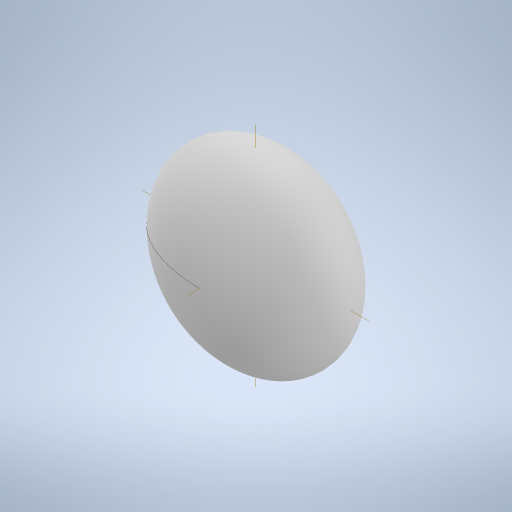
# Autodesk Inventor part: Ellipsoid
Saved by Autodesk Inventor 2023.1 (Build 271208000, 208)
## iProperties
Created: 2023-01-19
Part Number: Ellipsoid
Material: Generisch
Document SubType Name: Modeling
Designer: mehan
Density: 1 g/cm^3
Appearance: Vorgabe
Author: mehan
Autodesk Inventor part; units mm, degrees
ref_plane "YZ Plane" through (0, 0, 0) normal (1, 0, 0) x (0, 1, 0)
ref_plane "XZ Plane" through (0, 0, 0) normal (0, 1, 0) x (-1, 0, 0)
ref_plane "XY Plane" through (0, 0, 0) normal (0, 0, 1) x (1, 0, 0)
sketch "Skizze1" plane through (0, 0, 0) normal (0, 1, 0) x (-1, 0, 0)
  ellipse E0 centre (0, 0) end of major axis (75, 0) minor radius 45 (0, -45) -> (0, 45) ccw
  line L0 (0, 45) -> (0, -45)
  line L1 (0, 0) -> (75, 0) construction
  dimension "d4" = 90
  dimension "d5" = 75
  constraints: 4 end point, 1 coincident, 1 horizontal, 1 midpoint, 1 vertical, 5 other
  measures "d4" diameter of L0.start L1.start
  measures "d5" distance of L1.start L1.end
revolve "Umdrehung1" add sketch "Skizze1" angle 360 about axis through (0, 0, 45) along (0, 0, -1)
